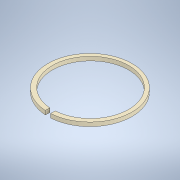
# Autodesk Inventor part: piston compression ring
Saved by Autodesk Inventor 2020 (Build 240168000, 168)
## iProperties
Created: 2020-08-04
Part Number: piston compression ring
Material: Generic
Document SubType Name: Modeling
Designer: benny
Density: 1 g/cm^3
Appearance: Default
Author: benny
Autodesk Inventor part; units mm, degrees
ref_plane "YZ Plane" through (0, 0, 0) normal (1, 0, 0) x (0, 1, 0)
ref_plane "XZ Plane" through (0, 0, 0) normal (0, 1, 0) x (-1, 0, 0)
ref_plane "XY Plane" through (0, 0, 0) normal (0, 0, 1) x (1, 0, 0)
sketch "Sketch1" plane through (0, 0, 0) normal (0, 1, 0) x (-1, 0, 0)
  circle A0 centre (0, 0.2173) radius 16
  point P0 (0, 0)
  dimension "d0" = 32
  constraints: 1 centre point
  measures "d0" diameter of A0
extrude "Extrusion1" add sketch "Sketch1" along normal blind 1.5
sketch "Sketch2" plane through (0, 1.5, 0.2173) normal (0, 1, 0) x (1, 0, 0)
  circle A0 centre (0, 0.2173) radius 14.5
  dimension "d3" = 29
  constraints: 1 centre point, 1 coincident
  measures "d3" diameter of A0
extrude "Extrusion2" cut sketch "Sketch2" against normal blind 1.5
sketch "Sketch3" plane through (0, 1.5, 0.2173) normal (0, 1, 0) x (1, 0, 0)
  line L0 (-1, -17.209) -> (1, -17.209)
  line L1 (1, -17.209) -> (1, -13.4717)
  line L2 (1, -13.4717) -> (-1, -13.4717)
  line L3 (-1, -13.4717) -> (-1, -17.209)
  line L4 (-1, -17.209) -> (1, -13.4717) construction
  line L5 (1, -17.209) -> (-1, -13.4717) construction
  point P0 (0, 0.2173)
  point P1 (0, -15.3403)
  dimension "d6" = 2
  constraints: 12 end point, 2 midpoint, 2 parallel, 1 horizontal, 1 perpendicular
  measures "d6" distance of L2.end L1.end
extrude "Extrusion3" cut sketch "Sketch3" against normal blind 1.5
body "Solid1"
